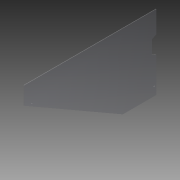
# Autodesk Inventor part: side panel
Saved by Autodesk Inventor 2015 SP1 (Build 190203100, 203)
## iProperties
Created: 2015-01-20
Part Number: side panel
Material: Generic
Document SubType Name: Modeling
Designer: Jarod
Density: 1 g/cm^3
Appearance: Default
Author: Jarod
Autodesk Inventor part; units mm, degrees
ref_plane "YZ Plane" through (0, 0, 0) normal (1, 0, 0) x (0, 1, 0)
ref_plane "XZ Plane" through (0, 0, 0) normal (0, 1, 0) x (-1, 0, 0)
ref_plane "XY Plane" through (0, 0, 0) normal (0, 0, 1) x (1, 0, 0)
sketch "Sketch1" plane through (0, 0, 0) normal (1, 0, 0) x (0, 1, 0)
  line L0 (0, 0) -> (-127, 0)
  line L1 (0, 0) -> (127, 0) construction
  line L2 (-227.417, 0) -> (-428.6358, 0)
  line L3 (0, 0) -> (0, 762)
  line L4 (0, 0) -> (762, 0) construction
  line L5 (0, 762) -> (-101.6, 762)
  line L6 (-101.6, 762) -> (-428.6358, 193.675)
  line L7 (-428.6358, 193.675) -> (-428.6358, 0)
  line L8 (-127, 0) -> (-137.521, 25.4)
  line L9 (-127, 0) -> (-99.5072, 0) construction
  line L10 (-137.521, 25.4) -> (-216.896, 25.4)
  line L11 (-216.896, 25.4) -> (-227.417, 0)
  dimension "d0" = 127
  dimension "d1" = 180
  dimension "d8" = 201.2188
  dimension "d10" = 762
  dimension "d11" = 90
  dimension "d13" = 90
  dimension "d14" = 90
  dimension "d18" = 112.5
  dimension "d19" = 79.375
  dimension "d20" = 112.5
  dimension "d21" = 112.5
  dimension "d22" = 25.4
  dimension "d23" = 0
  dimension "d35" = 101.6
  dimension "d36" = 193.675
  constraints: 24 end point, 5 horizontal, 3 equal length, 1 vertical
  measures "d0" distance of L0.start L0.end
  measures "d1" angle of L0 L1
  measures "d8" distance of L2.start L2.end
  measures "d10" distance of L0.start L3.end
  measures "d11" angle of L4 L3
  measures "d13" angle of L2 L7
  measures "d14" angle of L3 L5
  measures "d18" angle of L9 L8
  measures "d19" distance of L8.end L10.end
  measures "d20" angle of L2 L11
  measures "d21" angle of L10 L11
  measures "d22" distance from line of L0.start L10
  measures "d23" distance from line of L0.end L2
  measures "d35" distance of L3.end L5.end
  measures "d36" distance of L6.end L2.end
extrude "Extrusion1" add sketch "Sketch1" along normal blind 3.175
sketch "Sketch2" plane through (0, 0, 0) normal (-1, 0, 0) x (0, 0, 1)
  line L0 (0, 0) -> (0, -127) projected
  line L1 (0, -127) -> (25.4, -137.521) projected
  line L2 (25.4, -137.521) -> (25.4, -216.896) projected
  line L3 (25.4, -216.896) -> (0, -227.417) projected
  line L4 (0, -227.417) -> (0, -428.6358) projected
  line L5 (0, -428.6358) -> (193.675, -428.6358) projected
  line L6 (193.675, -428.6358) -> (762, -101.6) projected
  line L7 (762, -101.6) -> (762, 0) projected
  line L8 (762, 0) -> (0, 0) projected
  point P0 (12.7, -377.8358)
  point P1 (717.55, -111.125)
  dimension "d24" = 111.125
  dimension "d25" = 44.45
  dimension "d26" = 50.8
  dimension "d27" = 12.7
  measures "d24" distance from line of L8 point (717.55, -111.125)
  measures "d25" distance from line of L7 point (717.55, -111.125)
  measures "d26" distance from line of point (12.7, -377.836) L5
  measures "d27" distance from line of L4 point (12.7, -377.836)
hole "Hole1" at (0, -377.8358, 12.7) at (0, -111.125, 717.55) direction (1, 0, 0) diameter 6.35 end through all
body "Solid1"
